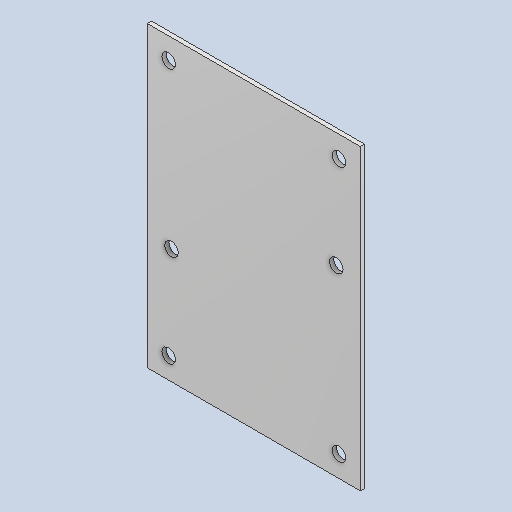
# Autodesk Inventor part: signal_combiner_plate
Saved by Autodesk Inventor 2023 (Build 270158000, 158)
## iProperties
Created: 2023-05-29
Part Number: signal_combiner_plate
Material: Aluminum
Document SubType Name: Sheet Metal
Designer: 310611102
Density: 2.7 g/cm^3
Sheet Metal Rule: Default_mm
Appearance: Satin
Author: 310611102
Autodesk Inventor part; units mm, degrees
ref_plane "YZ Plane" through (0, 0, 0) normal (1, 0, 0) x (0, 1, 0)
ref_plane "XZ Plane" through (0, 0, 0) normal (0, 1, 0) x (-1, 0, 0)
ref_plane "XY Plane" through (0, 0, 0) normal (0, 0, 1) x (1, 0, 0)
sketch "Sketch1" plane through (0, 0, 0) normal (0, 0, 1) x (1, 0, 0)
  line L0 (-25, 35) -> (25, 35)
  line L1 (25, 35) -> (25, -35)
  line L2 (25, -35) -> (-25, -35)
  line L3 (-25, -35) -> (-25, 35)
  line L4 (-25, 35) -> (25, -35) construction
  line L5 (25, 35) -> (-25, -35) construction
  circle A0 centre (-20, 30) radius 1.6
  line L6 (0, 0) -> (0, 8.6163)
  line L7 (0, 0) -> (6.049, 0)
  circle A1 centre (20, 30) radius 1.6
  circle A2 centre (-20, -30) radius 1.6
  circle A3 centre (20, -30) radius 1.6
  dimension "d0" = 50
  dimension "d1" = 70
  dimension "d12" = 3.2
  dimension "d13" = 5
  dimension "d18" = 5
  measures "d0" distance of L0.start L0.end
  measures "d1" distance of L0.end L1.end
  measures "d12" diameter of A0
  measures "d13" distance from line of L0 A0.centre
  measures "d18" distance from line of L3 A0.centre
extrude "Plate1" add sketch "Sketch1" along normal blind 1
sketch "Sketch2" plane through (0, 0, 1) normal (0, 0, 1) x (1, 0, 0)
  line L0 (22.55, 9.3405) -> (22.55, -9.3405)
  line L1 (22.55, -9.3405) -> (9.3405, -22.55)
  line L2 (9.3405, -22.55) -> (-9.3405, -22.55)
  line L3 (-9.3405, -22.55) -> (-22.55, -9.3405)
  line L4 (-22.55, -9.3405) -> (-22.55, 9.3405)
  line L5 (-22.55, 9.3405) -> (-9.3405, 22.55)
  line L6 (-9.3405, 22.55) -> (9.3405, 22.55)
  line L7 (9.3405, 22.55) -> (22.55, 9.3405)
  circle A0 centre (19.35, 8.015) radius 1.6
  line L8 (22.55, 9.3405) -> (-22.55, -9.3405)
  circle A1 centre (-19.35, -8.015) radius 1.6
  point P0 (0, 0)
  point P1 (0, 0)
  dimension "d3" = 45.1
  dimension "d4" = 3.2
  dimension "d5" = 3.2
  dimension "d8" = 360
  constraints: 18 end point, 2 centre point, 1 coincident, 1 point on line, 1 vertical, 22 other
  measures "d3" distance between parallel lines of L0 L4
  measures "d4" distance from line of L7 A0.centre
  measures "d5" diameter of A0
extrude "Extrusion1" cut sketch "Sketch2" against normal blind 10 contours L8 A0 | A0 L8 | A1 L8 | L8 A1
equation "\"d2\" = 厚度"
equation "\"折彎半徑\" = 厚度"
equation "\"折彎離隙寬度\" = 厚度"
equation "\"折彎離隙深度\" = 0.5 * 厚度"
equation "\"轉角離隙大小\" = 4 * 厚度"
equation "\"最小剩餘\" = 2 * 厚度"
equation "\"轉移半徑\" = 折彎半徑"
equation "\"Jacobi半徑大小\" = 折彎半徑"
equation "\"間隙大小\" = 厚度"
equation "\"厚度\" = 1"
body "Solid1"
